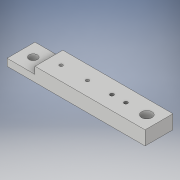
# Autodesk Inventor part: L17_TSI_005
Saved by Autodesk Inventor 2017 (Build 210142000, 142)
## iProperties
Created: 2017-03-02
Part Number: L17_TSI_005
Material: Generic
Document SubType Name: Modeling
Designer: coffmant
Density: 1 g/cm^3
Appearance: Default
Author: coffmant
Autodesk Inventor part; units mm, degrees
ref_plane "YZ Plane" through (0, 0, 0) normal (1, 0, 0) x (0, 1, 0)
ref_plane "XZ Plane" through (0, 0, 0) normal (0, 1, 0) x (-1, 0, 0)
ref_plane "XY Plane" through (0, 0, 0) normal (0, 0, 1) x (1, 0, 0)
sketch "Sketch1" plane through (0, 0, 0) normal (1, 0, 0) x (0, 1, 0)
  line L0 (0, 0) -> (12.7, 0)
  line L1 (12.7, 0) -> (12.7, -25.4)
  line L2 (12.7, -25.4) -> (0, -25.4)
  line L3 (0, -25.4) -> (0, 0)
  dimension "d0" = 12.7
  dimension "d1" = 25.4
  constraints: 8 end point, 2 parallel, 1 horizontal, 1 perpendicular
  measures "d0" distance between parallel lines of L3 L1
  measures "d1" distance between parallel lines of L0 L2
extrude "Extrusion1" add sketch "Sketch1" along normal blind 125.6538
sketch "Sketch3" plane through (0, 12.7, 0) normal (0, 1, 0) x (1, 0, 0)
  line L0 (0, 0) -> (125.6538, 0) projected
  line L1 (0, 25.4) -> (125.6538, 25.4) projected
  circle A0 centre (11.1125, 12.7) radius 6.35 projected
  circle A1 centre (114.5413, 12.7) radius 6.35 projected
  point P0 (36.5125, 12.7)
  point P1 (60.5125, 12.7)
  dimension "d13" = 25.4
  dimension "d14" = 12.7
  dimension "d16" = 24
  dimension "d36" = 25.4
  constraints: 1 horizontal alignment
  measures "d13" distance between parallel lines of L0 L1
  measures "d14" distance from line of L0 point (36.513, 12.7)
  measures "d16" distance of point (60.513, 12.7) point (36.513, 12.7)
  measures "d36" distance of A0.centre point (36.513, 12.7)
hole "Hole1" at (36.5125, 12.7, -12.7) at (60.5125, 12.7, -12.7) direction (0, -1, 0) diameter 3 end through all
sketch "Sketch5" plane through (0, 12.7, 0) normal (0, 1, 0) x (1, 0, 0)
  line L0 (0, 0) -> (125.6538, 0) projected
  line L1 (0, 25.4) -> (125.6538, 25.4) projected
  circle A0 centre (114.5413, 12.7) radius 6.35 projected
  point P0 (95.4913, 12.7)
  dimension "d26" = 12.7
  dimension "d27" = 25.4
  dimension "d28" = 19.05
  measures "d26" distance from line of L0 point (95.491, 12.7)
  measures "d27" distance between parallel lines of L0 L1
  measures "d28" distance of A0.centre point (95.491, 12.7)
hole "Hole2" at (95.4913, 12.7, -12.7) direction (0, -1, 0) diameter 3.302 end through all thread size "8-32 UNC" class "2B" standard "ANSI Unified Screw Threads"
sketch "Sketch12" plane through (0, 12.7, 0) normal (0, 1, 0) x (1, 0, 0)
  circle A0 centre (95.4913, 12.7) radius 1.651 projected
  circle A1 centre (36.5125, 12.7) radius 1.5 projected
  circle A2 centre (60.5125, 12.7) radius 1.5 projected
  line L0 (0, 0) -> (0, 25.4) projected
  line L1 (0, 0) -> (125.6538, 0) projected
  line L2 (125.6538, 25.4) -> (125.6538, 0) projected
  line L3 (0, 25.4) -> (125.6538, 25.4) projected
  point P0 (0, 0)
  point P1 (82.7913, 12.7)
  dimension "d77" = 12.7
  dimension "d78" = 12.7
  dimension "d79" = 12.7
  measures "d77" distance of A0.centre point (82.791, 12.7)
  measures "d78" distance from line of L1 A0.centre
  measures "d79" distance from line of L1 point (82.791, 12.7)
hole "Hole5" at (82.7913, 12.7, -12.7) direction (0, -1, 0) diameter 3.302 end through all thread size "8-32 UNC" class "2B" standard "ANSI Unified Screw Threads"
sketch "Sketch14" plane through (0, 12.7, 0) normal (0, 1, 0) x (1, 0, 0)
  circle A0 centre (82.7913, 12.7) radius 1.651 projected
  circle A1 centre (95.4913, 12.7) radius 1.651 projected
  circle A2 centre (36.5125, 12.7) radius 1.5 projected
  circle A3 centre (60.5125, 12.7) radius 1.5 projected
  line L0 (0, 0) -> (0, 25.4) projected
  line L1 (0, 0) -> (125.6538, 0) projected
  line L2 (125.6538, 25.4) -> (125.6538, 0) projected
  line L3 (0, 25.4) -> (125.6538, 25.4) projected
  point P0 (0, 0)
  point P1 (11.1125, 12.7)
hole "Hole7" at (11.1125, 12.7, -12.7) direction (0, -1, 0) diameter 7.62 end through all
sketch "Sketch15" plane through (0, 12.7, 0) normal (0, 1, 0) x (1, 0, 0)
  circle A0 centre (11.1125, 12.7) radius 3.81 projected
  circle A1 centre (82.7913, 12.7) radius 1.651 projected
  circle A2 centre (95.4913, 12.7) radius 1.651 projected
  circle A3 centre (36.5125, 12.7) radius 1.5 projected
  circle A4 centre (60.5125, 12.7) radius 1.5 projected
  line L0 (0, 0) -> (0, 25.4) projected
  line L1 (0, 0) -> (125.6538, 0) projected
  line L2 (125.6538, 25.4) -> (125.6538, 0) projected
  line L3 (0, 25.4) -> (125.6538, 25.4) projected
  circle A5 centre (114.5413, 12.7) radius 4.7625 projected
  point P0 (0, 0)
  constraints: 1 coincident
hole "Hole8" at (114.5413, 12.7, -12.7) direction (0, -1, 0) diameter 9.525 end through all
sketch "Sketch16" plane through (0, 12.7, 0) normal (0, 1, 0) x (1, 0, 0)
  circle A0 centre (114.5413, 12.7) radius 4.7625 projected
  circle A1 centre (11.1125, 12.7) radius 3.81 projected
  circle A2 centre (82.7913, 12.7) radius 1.651 projected
  circle A3 centre (95.4913, 12.7) radius 1.651 projected
  circle A4 centre (36.5125, 12.7) radius 1.5 projected
  circle A5 centre (60.5125, 12.7) radius 1.5 projected
  line L0 (0, 0) -> (0, 25.4) projected
  line L1 (0, 0) -> (125.6538, 0) projected
  line L2 (125.6538, 25.4) -> (125.6538, 0) projected
  line L3 (0, 25.4) -> (125.6538, 25.4) projected
  line L4 (0, 0) -> (125.6538, 0) projected
  line L5 (0, 0) -> (25.4, 0)
  line L6 (25.4, 0) -> (25.4, 25.4)
  line L7 (25.4, 25.4) -> (0, 25.4)
  line L8 (0, 25.4) -> (0, 0)
  dimension "d110" = 25.4
  constraints: 8 end point, 2 parallel, 1 horizontal, 1 perpendicular, 1 point on line
  measures "d110" distance between parallel lines of L0 L6
extrude "Extrusion7" cut sketch "Sketch16" against normal blind 6.35 contours L0 L3 L6 L1
equation "\"d14\" = 0.5 * d13"
equation "\"d26\" = 0.5 * d27"
equation "\"d79\" = d78"
body "Solid1"
